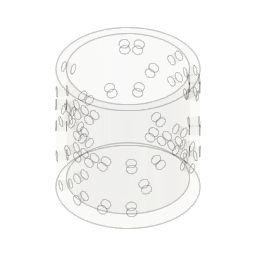
LET THE FLAMES SPREAD THE FIRE v9 (Autodesk Fusion 360 design; units mm, degrees)
Autodesk Fusion 360 part; units mm, degrees
note: some values were not read from the file. Chosen so that the rebuilt part matches the saved one: which bodies a step acts on.
sketch "Sketch1" plane through (0, 0, 0) normal (0, 0, 1) x (1, 0, 0)
  circle A0 centre (0, 0) radius 27.5
  dimension "d1" = 55
  constraint coincident A0.centre origin
  measures "d1" diameter of A0
extrude "Extrude1" add sketch "Sketch1" along normal blind 55 makes body 1
ref_plane "WorkPlane1" through (0, -27.5, 24.4489) normal (0, -1, 0) x (-1, 0, 0)
sketch "Sketch2" plane through (0, -27.5, 24.4489) normal (0, -1, 0) x (1, 0, 0)
  circle A0 centre (0, 13.0511) radius 3
  circle A1 centre (0, 23.0511) radius 3
  circle A2 centre (0, -6.9489) radius 3
  circle A3 centre (0, -16.9489) radius 3
  circle A4 centre (0, 3.0511) radius 3
  line L0 (27.5, -24.4489) -> (-27.5, -24.4489)
  dimension "d6" = 6
  dimension "d7" = 6
  dimension "d8" = 6
  dimension "d9" = 6
  dimension "d11" = 10
  dimension "d13" = 10
  dimension "d14" = 10
  dimension "d15" = 10
  dimension "d16" = 6
  dimension "d17" = 27.5
  measures "d6" diameter of A0
  measures "d7" diameter of A1
  measures "d8" diameter of A2
  measures "d9" diameter of A3
  measures "d11" distance of A2.centre A3.centre
  measures "d13" distance of A0.centre A1.centre
  measures "d14" distance of A2.centre A4.centre
  measures "d15" distance of A0.centre A4.centre
  measures "d16" diameter of A4
  measures "d17" distance of A4.centre L0
sketch "Sketch1 (2)" plane through (0, -27.5, 24.4489) normal (0, -1, 0) x (1, 0, 0) in component "Holes"
  circle A0 centre (0, 3.0511) radius 2
  circle A1 centre (0, 13.0511) radius 2
  circle A2 centre (0, 23) radius 2
  circle A3 centre (0, -6.9489) radius 2
  circle A4 centre (0, -16.9489) radius 2
  line L0 (27.5, -24.4489) -> (-27.5, -24.4489)
  point P0 (0, 3.0511)
  point P1 (0, -6.9489)
  point P2 (0, 23.0511)
  dimension "d18" = 4
  dimension "d19" = 4
  dimension "d20" = 4
  dimension "d21" = 4
  dimension "d22" = 4
  dimension "d23" = 10
  dimension "d24" = 10
  dimension "d25" = 10
  dimension "d26" = 10
  dimension "d27" = 27.5
  measures "d18" diameter of A0
  measures "d19" diameter of A3
  measures "d20" diameter of A4
  measures "d21" diameter of A1
  measures "d22" diameter of A2
  measures "d23" distance of P1 P0
  measures "d24" distance of A4.centre P1
  measures "d25" distance of A1.centre P0
  measures "d26" distance of A1.centre P2
  measures "d27" distance of P0 L0
extrude "Extrude1'" add sketch "Sketch1 (2)" against normal blind 10 separate body makes body 2 at (1.9975, -20.8333, 27.4003) makes body 3 at (1.9975, -20.8333, 17.4003) makes body 4 at (1.9975, -20.8333, 7.4003) makes body 5 at (1.9975, -20.8333, 37.4003) makes body 6 at (1.9975, -20.8333, 47.3492) in component "Holes"
pattern_circular "C-Pattern1" count 30 over 360 about axis through (0, 0, -27.5) along (0, 0, 1) of "Extrude1'" makes body 7 at (6.2854, -19.9628, 37.4003) makes body 8 at (10.2985, -18.2197, 37.4003) makes body 9 at (15.8148, -18.3815, 37.3009) makes body 10 at (19.2909, -14.6918, 37.3009) makes body 11 at (19.041, -8.6868, 37.4003) makes body 12 at (23.6011, -5.5682, 37.4003) makes body 13 at (20.928, -0.1911, 37.4003) makes body 14 at (20.5104, 4.1642, 37.4003) makes body 15 at (19.1964, 8.3376, 37.4003) makes body 16 at (19.9339, 13.8068, 37.3009) makes body 17 at (14.1456, 15.4247, 37.4003) makes body 18 at (10.6295, 18.0286, 37.4003) makes body 19 at (8.0115, 22.8868, 37.3009) makes body 20 at (3.078, 24.0523, 37.3009) makes body 21 at (-1.9975, 20.8333, 37.4003) makes body 22 at (-6.2854, 19.9628, 37.4003) makes body 23 at (-10.2985, 18.2197, 37.4003) makes body 24 at (-15.8148, 18.3815, 37.3009) makes body 25 at (-16.8188, 12.4558, 37.4003) makes body 26 at (-19.041, 8.6868, 37.4003) makes body 27 at (-23.6011, 5.5682, 37.4003) makes body 28 at (-20.928, 0.1911, 37.4003) makes body 29 at (-20.5104, -4.1642, 37.4003) makes body 30 at (-19.1964, -8.3376, 37.4003) makes body 31 at (-19.9339, -13.8068, 37.3009) makes body 32 at (-14.1456, -15.4247, 37.4003) makes body 33 at (-10.6295, -18.0286, 37.4003) makes body 34 at (-8.0115, -22.8868, 37.3009) makes body 35 at (-2.3776, -20.7934, 37.4003) makes body 36 at (6.2854, -19.9628, 17.4003) makes body 37 at (10.2985, -18.2197, 17.4003) makes body 38 at (15.8148, -18.3815, 17.3009) makes body 39 at (19.2909, -14.6918, 17.3009) makes body 40 at (19.041, -8.6868, 17.4003) makes body 41 at (23.6011, -5.5682, 17.4003) makes body 42 at (20.928, -0.1911, 17.4003) makes body 43 at (20.5104, 4.1642, 17.4003) makes body 44 at (19.1964, 8.3376, 17.4003) makes body 45 at (19.9339, 13.8068, 17.3009) makes body 46 at (14.1456, 15.4247, 17.4003) makes body 47 at (10.6295, 18.0286, 17.4003) makes body 48 at (8.0115, 22.8868, 17.3009) makes body 49 at (3.078, 24.0523, 17.3009) makes body 50 at (-1.9975, 20.8333, 17.4003) makes body 51 at (-6.2854, 19.9628, 17.4003) makes body 52 at (-10.2985, 18.2197, 17.4003) makes body 53 at (-15.8148, 18.3815, 17.3009) makes body 54 at (-16.8188, 12.4558, 17.4003) makes body 55 at (-19.041, 8.6868, 17.4003) makes body 56 at (-23.6011, 5.5682, 17.4003) makes body 57 at (-20.928, 0.1911, 17.4003) makes body 58 at (-20.5104, -4.1642, 17.4003) makes body 59 at (-19.1964, -8.3376, 17.4003) makes body 60 at (-19.9339, -13.8068, 17.3009) makes body 61 at (-14.1456, -15.4247, 17.4003) makes body 62 at (-10.6295, -18.0286, 17.4003) makes body 63 at (-8.0115, -22.8868, 17.3009) makes body 64 at (-2.3776, -20.7934, 17.4003) makes body 65 at (6.2854, -19.9628, 27.4003) makes body 66 at (10.2985, -18.2197, 27.4003) makes body 67 at (15.8148, -18.3815, 27.3009) makes body 68 at (19.2909, -14.6918, 27.3009) makes body 69 at (19.041, -8.6868, 27.4003) makes body 70 at (23.6011, -5.5682, 27.4003) makes body 71 at (20.928, -0.1911, 27.4003) makes body 72 at (20.5104, 4.1642, 27.4003) makes body 73 at (19.1964, 8.3376, 27.4003) makes body 74 at (19.9339, 13.8068, 27.3009) makes body 75 at (14.1456, 15.4247, 27.4003) makes body 76 at (10.6295, 18.0286, 27.4003) makes body 77 at (8.0115, 22.8868, 27.3009) makes body 78 at (3.078, 24.0523, 27.3009) makes body 79 at (-1.9975, 20.8333, 27.4003) makes body 80 at (-6.2854, 19.9628, 27.4003) makes body 81 at (-10.2985, 18.2197, 27.4003) makes body 82 at (-15.8148, 18.3815, 27.3009) makes body 83 at (-16.8188, 12.4558, 27.4003) makes body 84 at (-19.041, 8.6868, 27.4003) makes body 85 at (-23.6011, 5.5682, 27.4003) makes body 86 at (-20.928, 0.1911, 27.4003) makes body 87 at (-20.5104, -4.1642, 27.4003) makes body 88 at (-19.1964, -8.3376, 27.4003) makes body 89 at (-19.9339, -13.8068, 27.3009) makes body 90 at (-14.1456, -15.4247, 27.4003) makes body 91 at (-10.6295, -18.0286, 27.4003) makes body 92 at (-8.0115, -22.8868, 27.3009) makes body 93 at (-2.3776, -20.7934, 27.4003) makes body 94 at (6.9711, -23.2248, 7.3009) makes body 95 at (10.2985, -18.2197, 7.4003) makes body 96 at (15.8148, -18.3815, 7.3009) makes body 97 at (19.2909, -14.6918, 7.3009) makes body 98 at (19.041, -8.6868, 7.4003) makes body 99 at (23.6011, -5.5682, 7.4003) makes body 100 at (20.928, -0.1911, 7.4003) makes body 101 at (20.5104, 4.1642, 7.4003) makes body 102 at (19.1964, 8.3376, 7.4003) makes body 103 at (19.9339, 13.8068, 7.3009) makes body 104 at (14.1456, 15.4247, 7.4003) makes body 105 at (10.6295, 18.0286, 7.4003) makes body 106 at (8.0115, 22.8868, 7.3009) makes body 107 at (3.078, 24.0523, 7.3009) makes body 108 at (-1.9975, 20.8333, 7.4003) makes body 109 at (-6.9711, 23.2248, 7.3009) makes body 110 at (-10.2985, 18.2197, 7.4003) makes body 111 at (-15.8148, 18.3815, 7.3009) makes body 112 at (-16.8188, 12.4558, 7.4003) makes body 113 at (-19.041, 8.6868, 7.4003) makes body 114 at (-23.6011, 5.5682, 7.4003) makes body 115 at (-20.928, 0.1911, 7.4003) makes body 116 at (-20.5104, -4.1642, 7.4003) makes body 117 at (-19.1964, -8.3376, 7.4003) makes body 118 at (-19.9339, -13.8068, 7.3009) makes body 119 at (-14.1456, -15.4247, 7.4003) makes body 120 at (-10.6295, -18.0286, 7.4003) makes body 121 at (-8.0115, -22.8868, 7.3009) makes body 122 at (-3.078, -24.0523, 7.3009) makes body 123 at (6.2854, -19.9628, 47.3492) makes body 124 at (10.2985, -18.2197, 47.3492) makes body 125 at (15.8148, -18.3815, 47.2497) makes body 126 at (19.2909, -14.6918, 47.2497) makes body 127 at (19.041, -8.6868, 47.3492) makes body 128 at (23.6011, -5.5682, 47.3492) makes body 129 at (20.928, -0.1911, 47.3492) makes body 130 at (20.5104, 4.1642, 47.3492) makes body 131 at (19.1964, 8.3376, 47.3492) makes body 132 at (19.9339, 13.8068, 47.2497) makes body 133 at (14.1456, 15.4247, 47.3492) makes body 134 at (10.6295, 18.0286, 47.3492) makes body 135 at (8.0115, 22.8868, 47.2497) makes body 136 at (3.078, 24.0523, 47.2497) makes body 137 at (-1.9975, 20.8333, 47.3492) makes body 138 at (-6.2854, 19.9628, 47.3492) makes body 139 at (-10.2985, 18.2197, 47.3492) makes body 140 at (-15.8148, 18.3815, 47.2497) makes body 141 at (-16.8188, 12.4558, 47.3492) makes body 142 at (-19.041, 8.6868, 47.3492) makes body 143 at (-23.6011, 5.5682, 47.3492) makes body 144 at (-20.928, 0.1911, 47.3492) makes body 145 at (-20.5104, -4.1642, 47.3492) makes body 146 at (-19.1964, -8.3376, 47.3492) makes body 147 at (-19.9339, -13.8068, 47.2497) makes body 148 at (-14.1456, -15.4247, 47.3492) makes body 149 at (-10.6295, -18.0286, 47.3492) makes body 150 at (-8.0115, -22.8868, 47.2497) makes body 151 at (-2.3776, -20.7934, 47.3492) in component "Holes"
shell "Shell1" thickness 4 removed faces 1 at (-15.4646, -3.3405, 55) on bodies 1
combine "Combine1" operation cut target body 1 tool bodies 34 46 146 68 140 109 95 19 3 44 93 135 133 137 88 90 149 21 108 121 76 106 75 72 110 151 14 6 58 86 5 115 4 97 40 62 2 82 23 128 132 66 123 73 141 84 70 134 65 32 keep tools
component "Holes" placed x (1, 0, 0) y (0, 1, 0) z (0, 0, 1) at (0, 0, 0)
hidden bodies 4 5 6 7 8 9 10 11 12 13 15 16 17 18 20 22 24 25 26 27 28 29 30 31 33 35 36 37 38 39 41 42 43 45 47 48 49 50 51 52 53 54 55 56 57 59 60 61 63 64 67 69 71 74 77 78 79 80 81 83 85 87 89 91 92 94 96 98 99 100 101 102 103 104 105 107 111 112 113 114 116 117 118 119 120 122 124 125 126 127 129 130 131 136 138 139 142 143 144 145 147 148 150
equation "d5 = 6 mm"
equation "d6 = d5"
equation "d7 = d5"
equation "d8 = d5"
equation "d9 = d5"
equation "d11 = d14"
equation "d13 = d14"
equation "d15 = d14"
equation "d16 = d8"
equation "d17 = ( 55 / 2 ) * 1 mm"
equation "d19 = d18"
equation "d20 = d18"
equation "d21 = d18"
equation "d22 = d18"
equation "d24 = d23"
equation "d25 = d23"
equation "d26 = d23"
equation "d27 = ( 55 / 2 ) * 1 mm"
named bodies: "Let the flames spread the fire"
